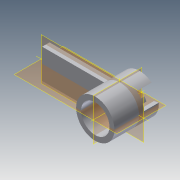
# Autodesk Inventor part: HbThumbProximalPhalanx01
Saved by Autodesk Inventor 2015 SP1 (Build 190203100, 203)
## iProperties
Created: 2015-09-12
Part Number: HbThumbProximalPhalanx01
Material: ABS プラスチック
Document SubType Name: Modeling
Designer: Yamaura
Density: 1.06 g/cm^3
Appearance: 滑らか - 白
Author: Yamaura
Autodesk Inventor part; units mm, degrees
sketch "スケッチ1" plane through (0, 0, 0) normal (0, 0, 1) x (1, 0, 0)
  circle A0 centre (0, 0) radius 5.75
  circle A1 centre (0, 0) radius 7.75
  dimension "d0" = 11.5
  dimension "d1" = 15.5
  constraints: 2 centre point, 2 coincident
  measures "d0" diameter of A0
  measures "d1" diameter of A1
extrude "押し出し1" add sketch "スケッチ1" along normal blind 10 and the other way blind 8 contours A0 | A1
sketch "スケッチ2" plane through (0, 0, 0) normal (0, 0, 1) x (1, 0, 0)
  line L0 (-30, 6) -> (0, 6)
  line L1 (0, 6) -> (0, -6)
  line L2 (0, -6) -> (-30, -6)
  line L3 (-30, -6) -> (-30, 6)
  point P0 (0, 0)
  dimension "d4" = 30
  dimension "d5" = 6
  dimension "d6" = 12
  constraints: 8 end point, 2 parallel, 1 horizontal, 1 midpoint, 1 perpendicular
  measures "d4" distance from line of L3 point (0, 0)
  measures "d5" distance from line of L0 point (0, 0)
  measures "d6" distance of L2.end L0.start
extrude "押し出し2" add sketch "スケッチ2" along normal mid plane 3
sketch "スケッチ5" plane through (0, 0, -8) normal (0, 0, -1) x (-1, 0, 0)
  circle A0 centre (0, 0) radius 5.75
  dimension "d21" = 11.5
  constraints: 1 centre point, 1 coincident
  measures "d21" diameter of A0
extrude "押し出し5" cut sketch "スケッチ5" against normal through all
sketch "スケッチ6" plane through (0, 0, -8) normal (0, 0, -1) x (-1, 0, 0)
  line L0 (11.4454, -3.8003) -> (-11.9713, 1.4586)
  line L1 (-11.9713, 1.4586) -> (-11.4454, 3.8003)
  line L2 (-11.4454, 3.8003) -> (11.9713, -1.4586)
  line L3 (11.9713, -1.4586) -> (11.4454, -3.8003)
  point P0 (0, 0)
  dimension "d24" = 1.2
  dimension "d34" = 2.4
  dimension "d35" = 12
  dimension "d36" = 24
  constraints: 8 end point, 2 parallel, 2 point on line, 1 perpendicular
  measures "d24" distance from line of L0 point (0, 0)
  measures "d34" distance of L0.end L1.end
  measures "d35" distance from line of L1 point (0, 0)
  measures "d36" distance of L2.start L2.end
extrude "押し出し6" cut sketch "スケッチ6" against normal blind 6
pattern_circular "円形状パターン2" count 2 over 30 about axis through (0, 0, -10) along (0, 0, 1) of "押し出し6"
move faces "移動1" translate (0, 0, 4.5) faces at (6.473, 2.8678, -8) (-6.0418, -3.6907, -8)
